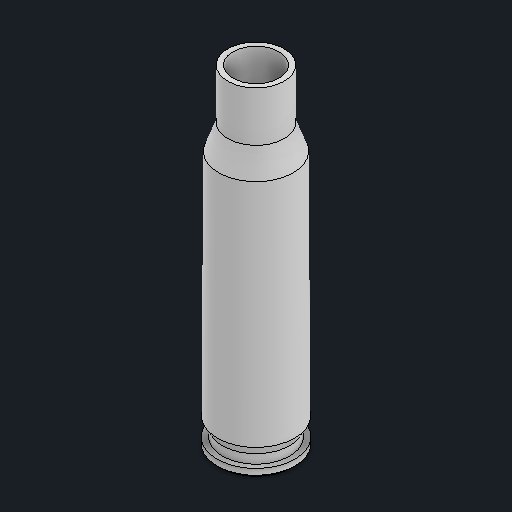
# Autodesk Inventor part: Part3
Saved by Autodesk Inventor 2025.1 (Build 291241020, 241B)
## iProperties
Created: 2025-05-15
Part Number: Part3
Material: Generic
Document SubType Name: Modeling
Designer: Joshua Eah
Density: 1 g/cm^3
Appearance: Default
Author: Joshua Eah
Autodesk Inventor part; units mm, degrees
sketch "Sketch1" plane through (0, 0, 0) normal (0, 1, 0) x (-1, 0, 0)
  circle A0 centre (0, 0) radius 6.007
  dimension "d0" = 12.014
  constraints: 1 centre point, 1 coincident
  measures "d0" diameter of A0
ref_plane "Work Plane1" through (0, 1.372, 0) normal (0, 1, 0) x (-1, 0, 0)
ref_plane "Work Plane2" through (0, 2.769, 0) normal (0, 1, 0) x (-1, 0, 0)
ref_plane "Work Plane3" through (0, 39.624, 0) normal (0, 1, 0) x (-1, 0, 0)
ref_plane "Work Plane4" through (0, 43.4848, 0) normal (0, 1, 0) x (-1, 0, 0)
ref_plane "Work Plane5" through (0, 51.181, 0) normal (0, 1, 0) x (-1, 0, 0)
ref_plane "Work Plane7" through (0, 4.166, 0) normal (0, 1, 0) x (-1, 0, 0)
sketch "Sketch2" plane through (0, 1.372, 0) normal (0, 1, 0) x (-1, 0, 0)
  circle A0 centre (0, 0) radius 5.1943
  dimension "d6" = 10.3886
  constraints: 1 centre point, 1 coincident
  measures "d6" diameter of A0
sketch "Sketch3" plane through (0, 2.769, 0) normal (0, 1, 0) x (-1, 0, 0)
  circle A0 centre (0, 0) radius 5.1943
  dimension "d7" = 10.3886
  constraints: 1 centre point, 1 coincident
  measures "d7" diameter of A0
sketch "Sketch4" plane through (0, 39.624, 0) normal (0, 1, 0) x (-1, 0, 0)
  circle A0 centre (0, 0) radius 5.7658
  dimension "d8" = 11.5316
  constraints: 1 centre point, 1 coincident
  measures "d8" diameter of A0
sketch "Sketch5" plane through (0, 43.4848, 0) normal (0, 1, 0) x (-1, 0, 0)
  circle A0 centre (0, 0) radius 4.3561
  dimension "d9" = 8.7122
  constraints: 1 centre point, 1 coincident
  measures "d9" diameter of A0
sketch "Sketch6" plane through (0, 51.181, 0) normal (0, 1, 0) x (-1, 0, 0)
  circle A0 centre (0, 0) radius 4.3561
  dimension "d10" = 8.7122
  constraints: 1 centre point, 1 coincident
  measures "d10" diameter of A0
sketch "Sketch8" plane through (0, 4.166, 0) normal (0, 1, 0) x (-1, 0, 0)
  circle A0 centre (0, 0) radius 5.969
  dimension "d37" = 11.938
  constraints: 1 centre point, 1 coincident
  measures "d37" diameter of A0
extrude "Extrusion1" add sketch "Sketch1" along normal up to surface (1.372 mm away)
extrude "Extrusion2" add sketch "Sketch2" along normal up to surface (1.397 mm away)
loft "Loft5" add profiles "Sketch8" section 1 edges at (5.1943, 2.769, 0)
loft "Loft6" add profiles "Sketch4" section 1 edges at (5.969, 4.166, 0)
loft "Loft7" add profiles "Sketch5" section 1 edges at (5.7658, 39.624, 0)
loft "Loft8" add profiles "Sketch6" section 1 edges at (4.3561, 43.4848, 0)
chamfer "Chamfer1" distance 0.458 angle 45 1 edges at (6.007, 0, 0)
shell "Shell1" thickness 0.8 removed faces 1 at (1.9818, 51.181, 0.7423)
body "Solid1"
